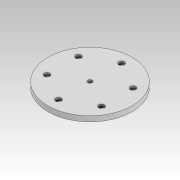
# Autodesk Inventor part: Flywheel
Saved by Autodesk Inventor 2020 (Build 240168000, 168)
## iProperties
Created: 2021-10-30
Part Number: Flywheel
Material: Generic
Document SubType Name: Modeling
Designer: DDeGo
Density: 1 g/cm^3
Appearance: Default
Author: DDeGo
Autodesk Inventor part; units mm, degrees
ref_plane "YZ Plane" through (0, 0, 0) normal (1, 0, 0) x (0, 1, 0)
ref_plane "XZ Plane" through (0, 0, 0) normal (0, 1, 0) x (-1, 0, 0)
ref_plane "XY Plane" through (0, 0, 0) normal (0, 0, 1) x (1, 0, 0)
sketch "Sketch1" plane through (0, 0, 0) normal (0, 0, 1) x (1, 0, 0)
  line L0 (0, 7) -> (0, 0) construction
  line L1 (0, 0) -> (1.05, 0) construction
  line L2 (1.05, 0) -> (1.05, 7)
  line L3 (1.05, 7) -> (0, 7) construction
  line L4 (1.05, 7) -> (20, 7)
  line L5 (2.8, 3) -> (2.5, 3)
  line L6 (2.5, 3) -> (2.5, 0)
  line L7 (2.5, 0) -> (1.05, 0)
  line L8 (20, 7) -> (20, 4.5)
  line L9 (20, 4.5) -> (2.8, 4.5)
  line L10 (2.8, 4.5) -> (2.8, 3)
  dimension "d0" = 2.5
  dimension "d1" = 1.05
  dimension "d3" = 0.3
  dimension "d4" = 3
  dimension "d9" = 1.5
  dimension "d10" = 20
  dimension "d11" = 2.5
  constraints: 22 end point, 7 perpendicular, 2 vertical, 1 horizontal
  measures "d0" distance between parallel lines of L0 L6
  measures "d1" distance between parallel lines of L0 L2
  measures "d3" distance of L5.start L5.end
  measures "d4" distance of L5.end L6.end
  measures "d9" distance of L9.end L5.start
  measures "d10" distance between parallel lines of L0 L8
  measures "d11" distance of L4.end L8.end
revolve "Revolution1" add sketch "Sketch1" angle 360 about axis through (0, 7, 0) along (0, -1, 0)
sketch "Sketch2" plane through (0, 7, 0) normal (0, 1, 0) x (1, 0, 0)
  line L0 (0, 0) -> (0, 15) construction
  circle A0 centre (0, 15) radius 1.35
  line L1 (0, 0) -> (-12.9904, 7.5) construction
  circle A1 centre (-12.9904, 7.5) radius 1.35
  line L2 (0, 0) -> (-12.9904, -7.5) construction
  circle A2 centre (-12.9904, -7.5) radius 1.35
  line L3 (0, 0) -> (0, -15) construction
  circle A3 centre (0, -15) radius 1.35
  line L4 (0, 0) -> (12.9904, -7.5) construction
  circle A4 centre (12.9904, -7.5) radius 1.35
  line L5 (0, 0) -> (12.9904, 7.5) construction
  circle A5 centre (12.9904, 7.5) radius 1.35
  dimension "d12" = 15
  dimension "d13" = 2.7
  dimension "d16" = 360
  constraints: 12 end point, 8 coincident, 6 centre point, 1 vertical, 29 other
  measures "d12" distance of L0.start L0.end
  measures "d13" diameter of A0
extrude "Extrusion1" cut sketch "Sketch2" against normal blind 10
sketch "Sketch3" plane through (0, 4.5, 0) normal (0, -1, 0) x (1, 0, 0)
  circle A0 centre (0, -15) radius 1.35 construction
  line L0 (-2.9445, -15) -> (-1.4722, -12.45)
  line L1 (-1.4722, -12.45) -> (1.4722, -12.45)
  line L2 (1.4722, -12.45) -> (2.9445, -15)
  line L3 (2.9445, -15) -> (1.4722, -17.55)
  line L4 (1.4722, -17.55) -> (-1.4722, -17.55)
  line L5 (-1.4722, -17.55) -> (-2.9445, -15)
  line L6 (11.5181, -10.05) -> (10.0459, -7.5)
  line L7 (10.0459, -7.5) -> (11.5181, -4.95)
  line L8 (11.5181, -4.95) -> (14.4626, -4.95)
  line L9 (14.4626, -4.95) -> (15.9349, -7.5)
  line L10 (15.9349, -7.5) -> (14.4626, -10.05)
  line L11 (14.4626, -10.05) -> (11.5181, -10.05)
  line L12 (14.4626, 4.95) -> (11.5181, 4.95)
  line L13 (11.5181, 4.95) -> (10.0459, 7.5)
  line L14 (10.0459, 7.5) -> (11.5181, 10.05)
  line L15 (11.5181, 10.05) -> (14.4626, 10.05)
  line L16 (14.4626, 10.05) -> (15.9349, 7.5)
  line L17 (15.9349, 7.5) -> (14.4626, 4.95)
  line L18 (2.9445, 15) -> (1.4722, 12.45)
  line L19 (1.4722, 12.45) -> (-1.4722, 12.45)
  line L20 (-1.4722, 12.45) -> (-2.9445, 15)
  line L21 (-2.9445, 15) -> (-1.4722, 17.55)
  line L22 (-1.4722, 17.55) -> (1.4722, 17.55)
  line L23 (1.4722, 17.55) -> (2.9445, 15)
  line L24 (-11.5181, 10.05) -> (-10.0459, 7.5)
  line L25 (-10.0459, 7.5) -> (-11.5181, 4.95)
  line L26 (-11.5181, 4.95) -> (-14.4626, 4.95)
  line L27 (-14.4626, 4.95) -> (-15.9349, 7.5)
  line L28 (-15.9349, 7.5) -> (-14.4626, 10.05)
  line L29 (-14.4626, 10.05) -> (-11.5181, 10.05)
  line L30 (-14.4626, -4.95) -> (-11.5181, -4.95)
  line L31 (-11.5181, -4.95) -> (-10.0459, -7.5)
  line L32 (-10.0459, -7.5) -> (-11.5181, -10.05)
  line L33 (-11.5181, -10.05) -> (-14.4626, -10.05)
  line L34 (-14.4626, -10.05) -> (-15.9349, -7.5)
  line L35 (-15.9349, -7.5) -> (-14.4626, -4.95)
  point P0 (0, 0)
  point P1 (12.9904, -7.5)
  point P2 (12.9904, -7.5)
  point P3 (12.9904, 7.5)
  point P4 (12.9904, 7.5)
  point P5 (0, 15)
  point P6 (0, 15)
  point P7 (-12.9904, 7.5)
  point P8 (-12.9904, 7.5)
  point P9 (-12.9904, -7.5)
  point P10 (-12.9904, -7.5)
  dimension "d20" = 5.1
  dimension "d23" = 360
  constraints: 72 end point, 6 coincident, 1 horizontal, 98 other
  measures "d20" distance between parallel lines of L1 L4
extrude "Extrusion2" cut sketch "Sketch3" against normal blind 1.5
chamfer "Chamfer2" distance 0.3 angle 45 1 edges at (-1.05, 0, 0)
body "Solid1"
